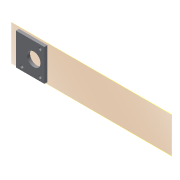
# Autodesk Inventor part: BallMount
Saved by Autodesk Inventor 2018 (Build 220112000, 112)
## iProperties
Created: 2019-02-16
Part Number: BallMount
Material: Generic
Document SubType Name: Modeling
Designer: ball
Density: 1 g/cm^3
Appearance: Default
Author: ball
Autodesk Inventor part; units mm, degrees
ref_plane "YZ Plane" through (0, 0, 0) normal (1, 0, 0) x (0, 1, 0)
ref_plane "XZ Plane" through (0, 0, 0) normal (0, 1, 0) x (-1, 0, 0)
ref_plane "XY Plane" through (0, 0, 0) normal (0, 0, 1) x (1, 0, 0)
ref_plane "Work Plane1" through (0, 0, 0) normal (0, 0, 1) x (1, 0, 0)
sketch "Sketch1" plane through (0, 0, 0) normal (0, 0, 1) x (1, 0, 0)
  line L0 (-192, 0) -> (-192, -43) construction
  line L1 (-192, -43) -> (0, -43) construction
  line L2 (-192, 0) -> (0, 0) construction
  line L3 (-153.9875, -0.508) -> (-153.9875, -42.492)
  line L4 (-153.9875, -42.492) -> (-191.492, -42.492)
  line L5 (-191.492, -42.492) -> (-191.492, -0.508)
  line L6 (-191.492, -0.508) -> (-153.9875, -0.508)
  circle A0 centre (-168, -21.5) radius 7.975 construction
  circle A1 centre (-168, -21.5) radius 8.89
  circle A2 centre (-184, -37.5) radius 2 construction
  circle A3 centre (-160, -37.5) radius 2 construction
  circle A4 centre (-160, -5.5) radius 2 construction
  circle A5 centre (-184, -37.5) radius 2.1844
  circle A6 centre (-160, -37.5) radius 2.1844
  circle A7 centre (-160, -5.5) radius 2.1844
extrude "Extrusion1" add sketch "Sketch1" along normal blind 4.064
body "Solid1"
